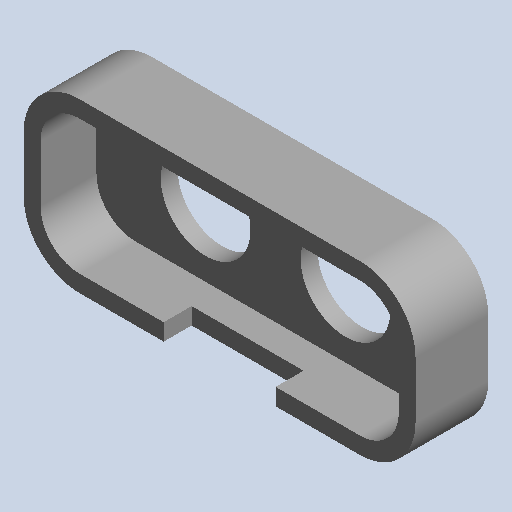
# Autodesk Inventor part: sensor_cover_ultrasonic
Saved by Autodesk Inventor 2026 (Build 300175050, 175E)
## iProperties
Part Number: sensor_cover_ultrasonic
Material: Generic
Document SubType Name: Modeling
Designer: Kartik
Mass: 9.73832 g
Surface Area: 73.723 cm^2
Volume: 9.73832 cm^3
Density: 1 g/cm^3
Appearance: Default
Author: Kartik
Autodesk Inventor part; units mm, degrees
ref_plane "YZ Plane" through (0, 0, 0) normal (1, 0, 0) x (0, 1, 0)
ref_plane "XZ Plane" through (0, 0, 0) normal (0, 1, 0) x (-1, 0, 0)
ref_plane "XY Plane" through (0, 0, 0) normal (0, 0, 1) x (1, 0, 0)
sketch "Sketch1" plane through (0, 0, 0) normal (0, 0, 1) x (1, 0, 0)
  line L0 (-35, 15) -> (35, 15)
  line L1 (35, 15) -> (35, -15)
  line L2 (35, -15) -> (-35, -15)
  line L3 (-35, -15) -> (-35, 15)
  point P0 (0, 0)
  dimension "d0" = 70
  dimension "d1" = 30
  dimension "d7" = 35
  dimension "d8" = 15
  constraints: 8 end point, 2 parallel, 1 horizontal, 1 perpendicular
  measures "d0" distance of L0.start L0.end
  measures "d1" distance of L2.end L0.start
  measures "d7" distance from line of L3 point (0, 0)
  measures "d8" distance from line of L0 point (0, 0)
extrude "Extrusion1" add sketch "Sketch1" along normal blind 3
sketch "Sketch2" plane through (0, 0, 3) normal (0, 0, 1) x (1, 0, 0)
  circle A0 centre (-12.5, 0) radius 8
  circle A1 centre (12.5, 0) radius 8
  line L0 (35, 15) -> (-35, 15) projected
  point P0 (0, 0)
  dimension "d4" = 16
  dimension "d5" = 16
  dimension "d6" = 25
  dimension "d9" = 12.5
  dimension "d10" = 15
  constraints: 2 centre point
  measures "d4" diameter of A0
  measures "d5" diameter of A1
  measures "d6" distance of A1.centre A0.centre
  measures "d9" distance of A0.centre point (0, 0)
  measures "d10" distance from line of L0 A0.centre
extrude "Extrusion2" cut sketch "Sketch2" against normal blind 3
fillet "Fillet1" radius 10 4 edges at (-35, 15, 1.5) (-35, -15, 1.5) (35, -15, 1.5) (35, 15, 1.5)
sketch "Sketch3" plane through (0, 0, 3) normal (0, 0, 1) x (1, 0, 0)
  line L0 (25, 15) -> (-25, 15) projected
  arc A0 (-25, 15) -> (-35, 5) centre (-25, 5) ccw projected
  line L1 (-35, 5) -> (-35, -5) projected
  arc A1 (-35, -5) -> (-25, -15) centre (-25, -5) ccw projected
  line L2 (-25, -15) -> (25, -15) projected
  arc A2 (25, -15) -> (35, -5) centre (25, -5) ccw projected
  line L3 (35, -5) -> (35, 5) projected
  arc A3 (35, 5) -> (25, 15) centre (25, 5) ccw projected
  line L4 (-25, 12) -> (25, 12)
  arc A4 (32, 5) -> (25, 12) centre (25, 5) ccw
  line L5 (32, 5) -> (32, -5)
  arc A5 (25, -12) -> (32, -5) centre (25, -5) ccw
  line L6 (25, -12) -> (-25, -12)
  arc A6 (-32, -5) -> (-25, -12) centre (-25, -5) ccw
  line L7 (-32, -5) -> (-32, 5)
  arc A7 (-25, 12) -> (-32, 5) centre (-25, 5) ccw
  point P0 (0, 0)
  dimension "d14" = 3
  constraints: 8 end point, 8 point on circle, 4 centre point, 7 other
  measures "d14" distance between parallel lines of L0 L4
extrude "Extrusion3" add sketch "Sketch3" along normal blind 10
sketch "Sketch4" plane through (-25, -12, 3) normal (0, 1, 0) x (1, 0, 0)
  line L0 (50, -10) -> (0, -10) construction
  line L1 (35, -10) -> (15, -10)
  line L2 (15, -10) -> (15, -5)
  line L3 (15, -5) -> (35, -5)
  line L4 (35, -5) -> (35, -10)
  point P0 (25, 3)
  point P1 (25, -10)
  point P2 (25, -10)
  dimension "d17" = 20
  dimension "d18" = 5
  dimension "d19" = 0
  constraints: 8 end point, 2 midpoint, 2 parallel, 1 horizontal, 1 perpendicular, 1 point on line
  measures "d17" distance of L2.end L3.end
  measures "d18" distance of L1.end L2.end
  measures "d19" distance of point (25, -10) point (25, -10)
extrude "Extrusion4" cut sketch "Sketch4" against normal blind 10
equation "\"d7\" = 0.5 * d0"
equation "\"d8\" = 0.5 * d1"
equation "\"d9\" = 0.5 * d6"
equation "\"d10\" = 0.5 * d1"
body "Solid1"
